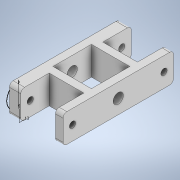
# Autodesk Inventor part: pullitens
Saved by Autodesk Inventor 2022 (Build 260153000, 153)
## iProperties
Created: 2022-03-11
Part Number: pullitens
Material: Genérico
Document SubType Name: Modeling
Designer: JK
Density: 1 g/cm^3
Appearance: Valor por defecto
Author: JK
Autodesk Inventor part; units mm, degrees
ref_plane "YZ Plane" through (0, 0, 0) normal (1, 0, 0) x (0, 1, 0)
ref_plane "XZ Plane" through (0, 0, 0) normal (0, 1, 0) x (-1, 0, 0)
ref_plane "XY Plane" through (0, 0, 0) normal (0, 0, 1) x (1, 0, 0)
sketch "Boceto1" plane through (0, 0, 0) normal (0, 1, 0) x (-1, 0, 0)
  line L0 (-10.15, 10.15) -> (10.15, 10.15)
  line L1 (10.15, 10.15) -> (10.15, -10.15)
  line L2 (10.15, -10.15) -> (-10.15, -10.15)
  line L3 (-10.15, -10.15) -> (-10.15, 10.15)
  line L4 (-10.15, 10.15) -> (10.15, -10.15) construction
  line L5 (10.15, 10.15) -> (-10.15, -10.15) construction
  line L6 (-14.15, 14.15) -> (14.15, 14.15)
  line L7 (14.15, 14.15) -> (14.15, -14.15)
  line L8 (14.15, -14.15) -> (-14.15, -14.15)
  line L9 (-14.15, -14.15) -> (-14.15, 14.15)
  line L10 (-14.15, 14.15) -> (14.15, -14.15) construction
  line L11 (14.15, 14.15) -> (-14.15, -14.15) construction
  point P0 (0, 0)
  dimension "d0" = 20.3
  dimension "d1" = 4
  constraints: 24 end point, 4 midpoint, 4 parallel, 3 perpendicular, 2 horizontal, 1 point on line
  measures "d0" distance of L0.start L0.end
  measures "d1" distance between parallel lines of L0 L6
extrude "Extrusión1" add sketch "Boceto1" along normal blind 15
sketch "Boceto3" plane through (0, 15, 0) normal (0, 1, 0) x (1, 0, 0)
  line L0 (-14.15, -29.15) -> (-8.15, -29.15)
  line L1 (-8.15, -29.15) -> (-8.15, 29.15)
  line L2 (-8.15, 29.15) -> (-14.15, 29.15)
  line L3 (-14.15, 29.15) -> (-14.15, -29.15)
  line L4 (14.15, 29.15) -> (10.15, 29.15)
  line L5 (10.15, 29.15) -> (10.15, -29.15)
  line L6 (10.15, -29.15) -> (14.15, -29.15)
  line L7 (14.15, -29.15) -> (14.15, 29.15)
  line L8 (14.15, 14.15) -> (-14.15, 14.15) projected
  line L9 (-14.15, 14.15) -> (-14.15, -14.15) projected
  line L10 (-14.15, -14.15) -> (14.15, -14.15) projected
  line L11 (14.15, -14.15) -> (14.15, 14.15) projected
  line L12 (10.15, -10.15) -> (-10.15, -10.15) projected
  line L13 (-10.15, -10.15) -> (-10.15, 10.15) projected
  line L14 (-10.15, 10.15) -> (10.15, 10.15) projected
  line L15 (10.15, 10.15) -> (10.15, -10.15) projected
  line L16 (10.15, 10.15) -> (10.15, -10.15) projected
  point P0 (-8.15, 14.15)
  point P1 (-8.15, -14.15)
  point P2 (10.15, 14.15)
  point P3 (10.15, -14.15)
  dimension "d10" = 6
  dimension "d11" = 15
  dimension "d12" = 15
  constraints: 16 end point, 4 collinear, 4 parallel, 2 horizontal, 2 perpendicular, 1 point on line
  measures "d10" distance between parallel lines of L3 L1
  measures "d11" distance between parallel lines of L10 L0
  measures "d12" distance between parallel lines of L2 L8
extrude "Extrusión2" add sketch "Boceto3" against normal up to surface (15 mm away) contours L3 L10 L1 L0 | L3 L2 L1 L8 | L10 L7 L6 L5 | L5 L4 L7 L8
sketch "Boceto4" plane through (-14.15, 15, -29.15) normal (-1, 0, 0) x (0, 0, 1)
  circle A0 centre (53.3, -7.5) radius 1.65
  circle A1 centre (5, -7.5) radius 1.65
  line L0 (15, -15) -> (15, 0) projected
  line L1 (0, 0) -> (58.3, 0) projected
  point P0 (29.15, -15)
  point P1 (43.3, 0)
  dimension "d15" = 3.3
  dimension "d16" = 3.3
  dimension "d23" = 10
  dimension "d24" = 10
  dimension "d25" = 7.5
  constraints: 2 centre point, 1 horizontal alignment
  measures "d15" diameter of A1
  measures "d16" diameter of A0
  measures "d23" horizontal distance of A0.centre point (43.3, 0)
  measures "d24" horizontal distance of L0.end A1.centre
  measures "d25" distance from line of A0.centre L1
extrude "Extrusión3" cut sketch "Boceto4" against normal through all
sketch "Boceto5" plane through (-14.15, 15, -29.15) normal (-1, 0, 0) x (0, 0, 1)
  circle A0 centre (53.3, -7.5) radius 1.65 projected
  circle A1 centre (53.3, -7.5) radius 6.5
  point P0 (29.15, -15)
  dimension "d22" = 13
  constraints: 1 centre point, 1 coincident
  measures "d22" diameter of A1
sketch "Boceto6" plane through (-14.15, 15, -29.15) normal (-1, 0, 0) x (0, 0, 1)
  circle A0 centre (29.15, -7.5) radius 2.7
  line L0 (58.3, -15) -> (0, -15) projected
  point P0 (29.15, -15)
  point P1 (29.15, -15)
  dimension "d26" = 5.4
  dimension "d27" = 7.5
  constraints: 1 centre point, 1 midpoint, 1 vertical alignment
  measures "d26" diameter of A0
  measures "d27" distance from line of L0 A0.centre
extrude "Extrusión4" cut sketch "Boceto6" against normal through all
fillet "Empalme1" radius 2 8 edges at (-11.15, 15, 29.15) (12.15, 15, 29.15) (12.15, 15, -29.15) (-11.15, 15, -29.15) (12.15, 0, 29.15) (-11.15, 0, 29.15) (12.15, 0, -29.15) (-11.15, 0, -29.15)
